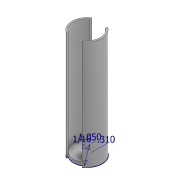
# Autodesk Inventor part: Sheath
Saved by Autodesk Inventor 2020.4 (Build 244396000, 396)
## iProperties
Created: 2022-05-28
Part Number: Sheath
Material: Generic
Document SubType Name: Modeling
Designer: david
Density: 1 g/cm^3
Appearance: Smooth - Medium Gray
Author: david
Autodesk Inventor part; units mm, degrees
ref_plane "YZ Plane" through (0, 0, 0) normal (1, 0, 0) x (0, 1, 0)
ref_plane "XZ Plane" through (0, 0, 0) normal (0, 1, 0) x (-1, 0, 0)
ref_plane "XY Plane" through (0, 0, 0) normal (0, 0, 1) x (1, 0, 0)
sketch "Sketch1" plane through (0, 0, 0) normal (0, 1, 0) x (-1, 0, 0)
  circle A0 centre (0, 0) radius 13.335
  line L0 (7.874, -12.676) -> (7.874, 12.676)
  line L1 (0, 0) -> (0, -4.5333)
  line L2 (-7.874, -12.676) -> (-7.874, 12.676)
  arc A1 (7.874, -12.676) -> (7.874, 12.676) centre (0, 0) ccw
  arc A2 (-7.874, 12.676) -> (-7.874, -12.676) centre (0, 0) ccw
  point P0 (-7.874, -10.7621)
  point P1 (-7.874, 10.7621)
  point P2 (7.874, 10.7621)
  point P3 (7.874, -10.7621)
  dimension "d0" = 26.67
  dimension "d6" = 7.874
  dimension "d11" = 1.5875
  constraints: 6 end point, 4 point on circle, 3 centre point, 2 coincident, 2 symmetric about line, 1 vertical
  measures "d0" diameter of A0
  measures "d6" distance between parallel lines of L1 L0
  measures "d11" radial gap between concentric circles of A1 A0
extrude "Extrusion1" add sketch "Sketch1" along normal blind 107.95 contours A0 L0 A1 | A0 L2 A2
extrude "Extrusion2" add sketch "Sketch1" along normal blind 3.175 contours A0 L0 | L0 A0 L2 | L2 A0
body "Solid1"
